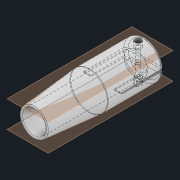
# Autodesk Inventor part: grip
Saved by Autodesk Inventor 2022 (Build 260153000, 153)
## iProperties
Created: 2024-04-29
Part Number: grip
Material: 一般
Document SubType Name: Modeling
Designer: gisen
Density: 1 g/cm^3
Appearance: 既定
Author: gisen
Autodesk Inventor part; units mm, degrees
ref_plane "YZ Plane" through (0, 0, 0) normal (1, 0, 0) x (0, 1, 0)
ref_plane "XY Plane" through (0, 0, 0) normal (0, 0, 1) x (1, 0, 0)
sketch "スケッチ1" plane through (0, 0, 0) normal (0, 1, 0) x (-1, 0, 0)
  line L0 (-10.7, 92) -> (-10.7, 0)
  line L1 (-10.7, 0) -> (0, 0)
  line L2 (0, 0) -> (0, -8)
  line L3 (0, -8) -> (-17, -8) construction
  line L4 (-17, -8) -> (-17, 42) construction
  line L5 (-16.9626, 42.8635) -> (-12.6963, 92.0864)
  arc A0 (-16.9626, 42.8635) -> (-17, 42) centre (-7, 42) ccw
  arc A1 (-10.7, 92) -> (-12.6963, 92.0864) centre (-11.7, 92) ccw
  circle A2 centre (0, -2) radius 1.65 construction
  circle A3 centre (0, -2) radius 6 construction
  circle A4 centre (-10.7, 0) radius 6.3 construction
  line L6 (-17, 42) -> (-17, 0)
  line L7 (-0.9394, -7.926) -> (-11.6864, -6.2223) construction
  arc A5 (-17, 0) -> (-11.6864, -6.2223) centre (-10.7, 0) ccw construction
  arc A6 (-0.9394, -7.926) -> (0, -8) centre (0, -2) ccw construction
  line L8 (0, -28.2306) -> (0, 113.2544) projected
  line L9 (-17, 0) -> (-17, -8)
  line L10 (-17, -8) -> (0, -8)
  dimension "d0" = 1
  dimension "d1" = 10
  dimension "d2" = 10.7
  dimension "d3" = 17
  dimension "d4" = 92
  dimension "d5" = 8
  dimension "d6" = 50
  dimension "d7" = 3.3
  dimension "d8" = 2
  constraints: 20 end point, 12 point on circle, 10 tangent, 7 centre point, 4 coincident, 4 perpendicular, 2 point on line, 1 collinear, 1 parallel, 1 vertical
  measures "d0" radius of A1
  measures "d1" radius of A0
  measures "d2" distance between parallel lines of L0 L2
  measures "d3" distance between parallel lines of L4 L2
  measures "d4" distance from line of A1.centre L1
  measures "d5" distance between parallel lines of L3 L1
  measures "d6" distance of L3.end L4.end
  measures "d7" diameter of A2
  measures "d8" distance from line of L1 A2.centre
revolve "回転1" add sketch "スケッチ1" angle 360 about axis through (0, 0, -10) along (0, 0, 1)
sketch "スケッチ2" plane through (0, 0, 0) normal (0, 1, 0) x (-1, 0, 0)
  circle A0 centre (0, -2) radius 1.65
  line L0 (10.7, 0) -> (-10.7, 0) projected
  point P0 (0, 0)
  dimension "d10" = 3.3
  dimension "d23" = 2
  constraints: 1 centre point, 1 coincident
  measures "d10" diameter of A0
  measures "d23" distance from line of point (0, -2) L0
extrude "押し出し1" cut sketch "スケッチ2" along normal through all both and the other way through all
sketch "スケッチ3" plane through (0, 0, 0) normal (1, 0, 0) x (0, 1, 0)
  line L0 (0, -10) -> (0, 0) construction
  line L1 (1, -10) -> (-1, -10)
  line L2 (-1, -10) -> (-0.4, 30.006)
  line L3 (0.4, 30.006) -> (1, -10)
  arc A0 (0.4, 30.006) -> (-0.4, 30.006) centre (0, 30) ccw
  dimension "d13" = 0.4
  dimension "d14" = 2
  dimension "d15" = 40
  constraints: 8 end point, 2 point on circle, 2 tangent, 1 centre point, 1 equal length, 1 horizontal, 1 midpoint, 1 vertical
  measures "d13" radius of A0
  measures "d14" distance of L1.start L1.end
  measures "d15" distance from line of L1 A0.centre
extrude "押し出し2" cut sketch "スケッチ3" along normal through all both and the other way through all
ref_plane "作業平面1" through (0, 12, 0) normal (0, 1, 0) x (-1, 0, 0)
ref_plane "作業平面2" through (0, -12, 0) normal (0, 1, 0) x (-1, 0, 0)
sketch "スケッチ4" plane through (0, 12, 0) normal (0, 1, 0) x (-1, 0, 0)
  circle A0 centre (0, -2) radius 2.9
  circle A1 centre (0, -2) radius 1.65 construction
  dimension "d20" = 5.8
  constraints: 1 centre point, 1 concentric
  measures "d20" diameter of A0
extrude "押し出し3" cut sketch "スケッチ4" along normal through all
sketch "スケッチ5" plane through (0, -12, 0) normal (0, 1, 0) x (-1, 0, 0)
  line L0 (-1.5877, -4.75) -> (-3.1754, -2)
  line L1 (-3.1754, -2) -> (-1.5877, 0.75)
  line L2 (-1.5877, 0.75) -> (1.5877, 0.75)
  line L3 (1.5877, 0.75) -> (3.1754, -2)
  line L4 (3.1754, -2) -> (1.5877, -4.75)
  line L5 (1.5877, -4.75) -> (-1.5877, -4.75)
  point P0 (0, 0)
  point P1 (0, -2)
  point P2 (0, -2)
  dimension "d24" = 5.5
  constraints: 12 end point, 1 coincident, 1 horizontal, 13 other
  measures "d24" distance between parallel lines of L5 L2
extrude "押し出し4" cut sketch "スケッチ5" against normal through all
fillet "フィレット1" radius 2 2 edges at (0, 17, -8) (0, -17, -8)
equation "\"d19\" = -d18"
equation "\"d18\" = 12"
